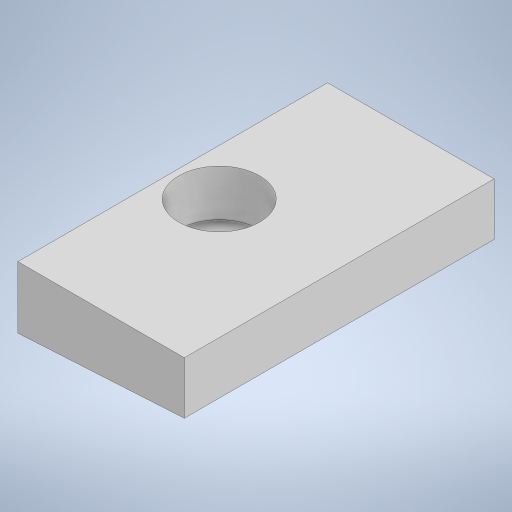
# Autodesk Inventor part: opaska_test
Saved by Autodesk Inventor 2024 (Build 280153000, 153)
## iProperties
Created: 2023-11-08
Part Number: opaska_test
Material: Generic
Document SubType Name: Modeling
Designer: Piotrek
Density: 1 g/cm^3
Appearance: Default
Author: Piotrek
Autodesk Inventor part; units mm, degrees
ref_plane "YZ Plane" through (0, 0, 0) normal (1, 0, 0) x (0, 1, 0)
ref_plane "XZ Plane" through (0, 0, 0) normal (0, 1, 0) x (-1, 0, 0)
ref_plane "XY Plane" through (0, 0, 0) normal (0, 0, 1) x (1, 0, 0)
sketch "Sketch1" plane through (0, 0, 0) normal (0, 1, 0) x (-1, 0, 0)
  line L0 (0, 0) -> (35, 0)
  line L1 (35, 0) -> (35, -20)
  line L2 (35, -20) -> (0, -20)
  line L3 (0, -20) -> (0, 0)
  dimension "d0" = 35
  dimension "d1" = 20
  constraints: 8 end point, 2 parallel, 1 horizontal, 1 perpendicular
  measures "d0" distance of L1.end L2.end
  measures "d1" distance of L0.end L1.end
extrude "Extrusion1" add sketch "Sketch1" along normal blind 2
sketch "Sketch2" plane through (0, 2, 0) normal (0, 1, 0) x (1, 0, 0)
  line L0 (-35, 20) -> (-35, 0) projected
  line L1 (-35, 10) -> (-32, 10)
  circle A0 centre (-32, 10) radius 2.6
  point P0 (0, 0)
  dimension "d4" = 3
  dimension "d5" = 5.2
  constraints: 2 end point, 1 centre point, 1 coincident, 1 horizontal, 1 midpoint
  measures "d4" distance of L1.start L1.end
  measures "d5" diameter of A0
extrude "Extrusion2" cut sketch "Sketch2" against normal blind 2
sketch "Sketch3" plane through (-35, 0, 0) normal (0, 0, 1) x (1, 0, 0)
  line L0 (35, 0) -> (0, 0) projected
  line L1 (0, 0) -> (0, -2)
  line L2 (0, -2) -> (35, 0)
  dimension "d8" = 2
  constraints: 4 end point, 1 vertical
  measures "d8" distance of L0.end L1.end
extrude "Extrusion3" add sketch "Sketch3" against normal up to surface (20 mm away)
sketch "Sketch4" plane through (0, 2, 0) normal (1, 0, 0) x (0, 0, -1)
  line L0 (0, -2) -> (20, -2) projected
  line L1 (0, -2) -> (20, -2)
  line L2 (20, -2) -> (20, 6.5769)
  line L3 (20, 6.5769) -> (0, 6.5769)
  line L4 (0, 6.5769) -> (0, -2)
  constraints: 8 end point, 2 parallel, 1 horizontal, 1 perpendicular
extrude "Extrusion4" cut sketch "Sketch4" against normal blind 23.75
sketch "Sketch5" plane through (0, 0, 0) normal (0, 1, 0) x (1, 0, 0)
  line L0 (-23.75, 20) -> (-35, 20) projected
  line L1 (-23.75, 20) -> (0, 20)
  line L2 (0, 20) -> (0, 0)
  line L3 (0, 0) -> (-23.75, 0)
  line L4 (-23.75, 0) -> (-23.75, 20)
  constraints: 8 end point, 2 parallel, 1 horizontal, 1 perpendicular
extrude "Extrusion5" cut sketch "Sketch5" against normal through all
sketch "Sketch6" plane through (-23.75, 2, 0) normal (1, 0, 0) x (0, 0, -1)
  line L0 (20, -4) -> (20, 0) projected
  line L1 (20, 0) -> (0, 0)
  line L2 (0, 0) -> (0, -8.1158)
  line L3 (0, -8.1158) -> (20, -8.1158)
  line L4 (20, -8.1158) -> (20, 0)
  point P0 (0, -2)
  constraints: 8 end point, 2 parallel, 1 horizontal, 1 perpendicular
extrude "Extrusion6" cut sketch "Sketch6" against normal blind 0.5
sketch "Sketch7" plane through (-32, 0, -10) normal (0, 1, 0) x (1, 0, 0)
  circle A0 centre (0, 0) radius 2.6
  point P0 (32, -10)
  dimension "d19" = 5.2
  constraints: 1 centre point
  measures "d19" diameter of A0
extrude "Extrusion7" cut sketch "Sketch7" against normal blind 1
body "Solid1"
